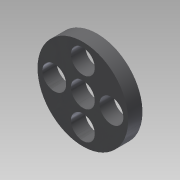
# Autodesk Inventor part: CounterArm
Saved by Autodesk Inventor 2014 (Build 180170000, 170)
## iProperties
Created: 2014-03-07
Part Number: CounterArm
Material: Générique
Document SubType Name: Modeling
Designer: Grégoire
Density: 1 g/cm^3
Appearance: Par défaut
Author: Grégoire
Autodesk Inventor part; units mm, degrees
ref_plane "YZ Plane" through (0, 0, 0) normal (1, 0, 0) x (0, 1, 0)
ref_plane "XZ Plane" through (0, 0, 0) normal (0, 1, 0) x (-1, 0, 0)
ref_plane "XY Plane" through (0, 0, 0) normal (0, 0, 1) x (1, 0, 0)
sketch "Esquisse1" plane through (0, 0, 0) normal (0, 1, 0) x (-1, 0, 0)
  circle A0 centre (0, 0) radius 9.5
  circle A1 centre (0, 0) radius 2.5
  line L0 (0, 9.5) -> (0, -9.5) construction
  line L1 (-9.5, 0) -> (9.5, 0) construction
  circle A2 centre (0, -6) radius 2.5
  circle A3 centre (0, 6) radius 2.5
  circle A4 centre (0, 0) radius 2.5
  circle A5 centre (6, 0) radius 2.5
  circle A6 centre (-6, 0) radius 2.5
  circle A7 centre (0, 0) radius 2.5
  dimension "d0" = 19
  dimension "d1" = 5
  dimension "d4" = 6
  dimension "d7" = 6
  dimension "d12" = 6
  dimension "d15" = 6
  constraints: 8 centre point, 4 end point, 4 point on circle, 2 coincident, 2 horizontal, 2 vertical, 1 perpendicular, 12 other
  measures "d0" diameter of A0
  measures "d1" diameter of A1
  measures "d4" distance of A1.centre A2.centre
  measures "d7" distance of A1.centre A3.centre
  measures "d12" distance of A1.centre A5.centre
  measures "d15" distance of A1.centre A6.centre
extrude "Extrusion1" add sketch "Esquisse1" along normal blind 3
